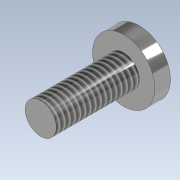
# Autodesk Inventor part: ネジ超低頭M3L8
Saved by Autodesk Inventor 2020.2 (Build 242310000, 310)
## iProperties
Created: 2020-05-25
Part Number: ネジ超低頭M3L8
Material: 鋼、高強度、低合金
Document SubType Name: Modeling
Designer: aoyama
Density: 7.85 g/cm^3
Appearance: 鋼 - つや出し
Author: aoyama
Autodesk Inventor part; units mm, degrees
ref_plane "YZ Plane" through (0, 0, 0) normal (1, 0, 0) x (0, 1, 0)
ref_plane "XZ Plane" through (0, 0, 0) normal (0, 1, 0) x (-1, 0, 0)
ref_plane "XY Plane" through (0, 0, 0) normal (0, 0, 1) x (1, 0, 0)
sketch "スケッチ1" plane through (0, 0, 0) normal (0, 0, 1) x (1, 0, 0)
  circle A0 centre (0, 0) radius 1.5
  circle A1 centre (0, 0) radius 3
  dimension "d0" = 3
  dimension "d1" = 6
  constraints: 2 centre point, 2 coincident
  measures "d0" diameter of A0
  measures "d1" diameter of A1
extrude "押し出し1" add sketch "スケッチ1" along normal blind 8 contours A0
extrude "押し出し2" add sketch "スケッチ1" against normal blind 1.5 contours A0 | A1
thread "ねじ1" size "M3x0.5" class "6g" standard "ANSI Metric M Profile" length 44.8
sketch "スケッチ2" plane through (0, 0, -1.5) normal (0, 0, -1) x (-1, 0, 0)
  circle A0 centre (0, 0) radius 3 projected
  line L0 (-0.75, 0.433) -> (0, 0.866)
  line L1 (0, 0.866) -> (0.75, 0.433)
  line L2 (0.75, 0.433) -> (0.75, -0.433)
  line L3 (0.75, -0.433) -> (0, -0.866)
  line L4 (0, -0.866) -> (-0.75, -0.433)
  line L5 (-0.75, -0.433) -> (-0.75, 0.433)
  dimension "d8" = 1.5
  constraints: 12 end point, 1 coincident, 1 vertical, 13 other
  measures "d8" distance between parallel lines of L3 L0
extrude "押し出し3" cut sketch "スケッチ2" against normal blind 2 contours L0 L1 L2 L3 L4 L5
fillet "フィレット1" radius 0.2 6 edges at (0.375, 0.6495, 0.5) (0.75, 0, 0.5) (0.375, -0.6495, 0.5) (-0.375, -0.6495, 0.5) (-0.75, 0, 0.5) (-0.375, 0.6495, 0.5)
